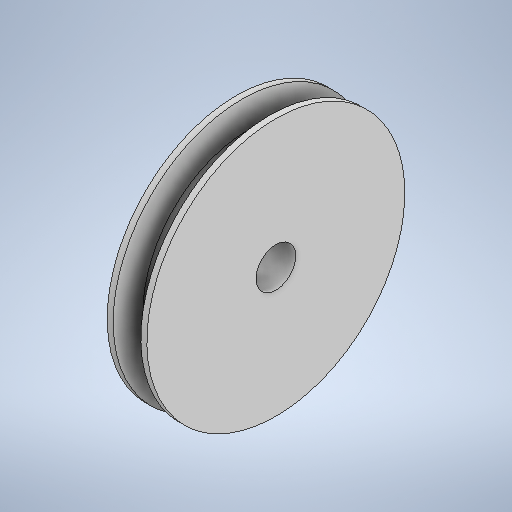
# Autodesk Inventor part: kolo
Saved by Autodesk Inventor 2025 (Build 290162000, 162)
## iProperties
Created: 2025-05-31
Part Number: kolo
Material: Ogólny
Document SubType Name: Modeling
Designer: tjaku
Density: 1 g/cm^3
Appearance: Domyślna
Author: tjaku
Autodesk Inventor part; units mm, degrees
ref_plane "YZ Plane" through (0, 0, 0) normal (1, 0, 0) x (0, 1, 0)
ref_plane "XZ Plane" through (0, 0, 0) normal (0, 1, 0) x (-1, 0, 0)
ref_plane "XY Plane" through (0, 0, 0) normal (0, 0, 1) x (1, 0, 0)
sketch "Szkic1" plane through (0, 0, 0) normal (0, 0, 1) x (1, 0, 0)
  line L0 (0, 0) -> (10, 0)
  line L1 (10, 0) -> (-10, 0)
  line L2 (-10, 0) -> (-10, 65)
  line L3 (10, 0) -> (10, 65)
  line L4 (-10, 65) -> (-10, 53)
  line L5 (10, 65) -> (7, 65)
  line L6 (-10, 65) -> (-7, 65)
  line L7 (4, 53) -> (-4, 53)
  line L8 (-7, 65) -> (-4, 53)
  line L9 (4, 53) -> (7, 65)
  point P0 (2, 53)
  dimension "d2" = 65
  dimension "d4" = 12
  dimension "d5" = 6
  dimension "d17" = 3
  dimension "d18" = 3
  constraints: 20 end point, 3 horizontal, 2 point on line, 1 perpendicular, 1 vertical
  measures "d2" distance of L1.end L2.end
  measures "d4" distance of L2.end L4.end
  measures "d5" distance of L4.end L7.end
  measures "d17" distance of L3.end L5.end
  measures "d18" distance of L2.end L6.end
revolve "Obrót1" add sketch "Szkic1" angle 360 about axis through (10, 0, 0) along (-1, 0, 0)
sketch "Szkic2" plane through (10, 0, 0) normal (1, 0, 0) x (0, 0, -1)
  circle A0 centre (0, 0) radius 10
  dimension "d8" = 20
  constraints: 1 centre point, 1 coincident
  measures "d8" diameter of A0
extrude "Wyciągnięcie proste1" cut sketch "Szkic2" against normal blind 100
